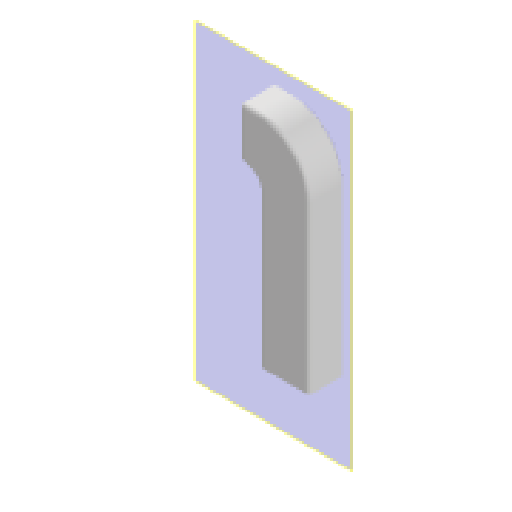
# Autodesk Inventor part: lock-arm
Saved by Autodesk Inventor 2024 (Build 280153000, 153)
## iProperties
Created: 2023-09-16
Part Number: lock-arm
Material: Generic
Document SubType Name: Modeling
Designer: draev
Density: 1 g/cm^3
Appearance: Default
Author: draev
Autodesk Inventor part; units mm, degrees
ref_plane "YZ Plane" through (0, 0, 0) normal (1, 0, 0) x (0, 1, 0)
ref_plane "XZ Plane" through (0, 0, 0) normal (0, 1, 0) x (-1, 0, 0)
ref_plane "XY Plane" through (0, 0, 0) normal (0, 0, 1) x (1, 0, 0)
ref_plane "Work Plane1" through (-0.7162, 26.4872, 4) normal (0, 0, -1) x (-1, 0, 0)
sketch "Sketch1" plane through (-0.7162, 26.4872, 4) normal (0, 0, -1) x (-1, 0, 0)
  arc A0 (-5.7162, 13.5128) -> (-20.7162, -1.4872) centre (-5.7162, -1.4872) ccw projected
  line L0 (-20.7162, -1.4872) -> (-20.7162, -49.4872) projected
  line L1 (-20.7162, -51.4872) -> (-20.7162, -49.4872) projected
  line L2 (-2, 13.5128) -> (-5.7162, 13.5128) projected
  line L3 (0, 13.5128) -> (-2, 13.5128) projected
  line L4 (-6.7162, -47.9738) -> (-6.7162, -5.4872)
  line L5 (-1.7162, -0.4872) -> (-1, -0.4872)
  arc A1 (-1.7162, -0.4872) -> (-6.7162, -5.4872) centre (-1.7162, -5.4872) ccw
  line L6 (-6.7162, -47.9738) -> (-20.7162, -47.9738)
  line L7 (-1, 13.5128) -> (-1, -0.4872)
  point P0 (-0.7162, -26.4872)
  dimension "d2" = 5
  constraints: 8 end point, 3 perpendicular, 2 point on circle, 2 tangent, 1 centre point, 1 midpoint, 1 point on line
  measures "d2" radius of A1
extrude "Extrusion1" add sketch "Sketch1" against normal blind 10
fillet "Fillet1" radius 1 14 edges at (3.1419, 40, 14) (0.7838, 40, 14) (20, 1.7567, 14) (15.6066, 35.6066, 14) (15.6066, 35.6066, 4) (3.1419, 40, 4) (0.7838, 40, 4) (20, 1.7567, 4) (6, -0.2433, 14) (0.6419, 26, 14) (4.5355, 24.5355, 14) (4.5355, 24.5355, 4) (0.6419, 26, 4) (6, -0.2433, 4)
fillet "Fillet2" radius 1 8 edges at (0.2838, 26.2929, 13.7071) (0.2838, 26, 9) (0.2838, 26.2929, 4.2929) (0.2838, 33, 4) (0.2838, 39.7071, 4.2929) (0.2838, 40, 9) (0.2838, 39.7071, 13.7071) (0.2838, 33, 14)
sketch "Sketch2" plane through (-0.7162, 26.4872, 14) normal (0, 0, 1) x (1, 0, 0)
  circle A0 centre (13.7162, -41.9738) radius 1.75
  line L0 (7.7162, -47.9738) -> (19.7162, -47.9738) projected
  line L1 (20.7162, -47.9738) -> (20.7162, -1.4872) projected
  point P0 (0.7162, -26.4872)
  dimension "d7" = 6
  dimension "d8" = 3.5
  dimension "d9" = 7
  constraints: 1 centre point
  measures "d7" distance from line of L0 A0.centre
  measures "d8" diameter of A0
  measures "d9" distance from line of L1 A0.centre
extrude "Extrusion2" cut sketch "Sketch2" against normal up to next
body "Solid1"
